Autodesk Inventor part; units mm, degrees
(part 2 of 2)
sketch "Sketch18" plane through (0, 0, 6.35) normal (0, 0, 1) x (1, 0, 0)
  line L0 (518.16, 78.74) -> (525.78, 78.74) construction
  line L1 (525.78, 78.74) -> (525.78, 162.56) construction
  line L2 (525.78, 162.56) -> (518.16, 162.56) construction
  line L3 (518.16, 162.56) -> (518.16, 193.04) construction
  line L4 (518.16, 193.04) -> (525.78, 193.04) construction
  line L5 (525.78, 193.04) -> (525.78, 276.86) construction
  line L6 (525.78, 276.86) -> (518.16, 276.86) construction
  line L7 (518.16, 276.86) -> (518.16, 307.34) construction
  line L8 (518.16, 307.34) -> (525.78, 307.34) construction
  line L9 (525.78, 307.34) -> (525.78, 355.6) construction
  line L10 (525.78, 355.6) -> (464.36, 355.6) construction
  line L11 (464.36, 355.6) -> (464.36, 347.98) construction
  line L12 (464.36, 347.98) -> (436.42, 347.98) construction
  line L13 (436.42, 347.98) -> (436.42, 355.6) construction
  line L14 (436.42, 355.6) -> (276.86, 355.6) construction
  line L15 (276.86, 355.6) -> (276.86, 347.98) construction
  line L16 (276.86, 347.98) -> (248.92, 347.98) construction
  line L17 (248.92, 347.98) -> (248.92, 355.6) construction
  line L18 (248.92, 355.6) -> (89.36, 355.6) construction
  line L19 (89.36, 355.6) -> (89.36, 347.98) construction
  line L20 (89.36, 347.98) -> (61.42, 347.98) construction
  line L21 (61.42, 347.98) -> (61.42, 355.6) construction
  line L22 (61.42, 355.6) -> (0, 355.6) construction
  line L23 (0, 355.6) -> (0, 307.34) construction
  line L24 (0, 307.34) -> (7.62, 307.34) construction
  line L25 (7.62, 307.34) -> (7.62, 276.86) construction
  line L26 (7.62, 276.86) -> (0, 276.86) construction
  line L27 (0, 276.86) -> (0, 193.04) construction
  line L28 (0, 193.04) -> (7.62, 193.04) construction
  line L29 (7.62, 193.04) -> (7.62, 162.56) construction
  line L30 (7.62, 162.56) -> (0, 162.56) construction
  line L31 (0, 162.56) -> (0, 78.74) construction
  line L32 (0, 78.74) -> (7.62, 78.74) construction
  line L33 (7.62, 78.74) -> (7.62, 48.26) construction
  line L34 (7.62, 48.26) -> (0, 48.26) construction
  line L35 (0, 48.26) -> (0, 0) construction
  line L36 (0, 0) -> (7.62, 0) construction
  line L37 (7.62, 0) -> (7.62, -79.375) construction
  line L38 (7.62, -79.375) -> (0, -79.375) construction
  line L39 (0, -79.375) -> (0, -104.775) construction
  line L40 (0, -104.775) -> (7.62, -104.775) construction
  line L41 (7.62, -104.775) -> (7.62, -177.8) construction
  line L42 (7.62, -177.8) -> (50.8, -177.8) construction
  line L43 (50.8, -177.8) -> (50.8, -185.42) construction
  line L44 (50.8, -185.42) -> (76.2, -185.42) construction
  line L45 (76.2, -185.42) -> (76.2, -177.8) construction
  line L46 (76.2, -177.8) -> (177.8, -177.8) construction
  line L47 (177.8, -177.8) -> (177.8, -185.42) construction
  line L48 (177.8, -185.42) -> (203.2, -185.42) construction
  line L49 (203.2, -185.42) -> (203.2, -177.8) construction
  line L50 (203.2, -177.8) -> (242.89, -177.8) construction
  line L51 (242.89, -177.8) -> (242.89, -127.8) construction
  line L52 (242.89, -127.8) -> (282.89, -127.8) construction
  line L53 (282.89, -127.8) -> (282.89, -177.8) construction
  line L54 (282.89, -177.8) -> (322.58, -177.8) construction
  line L55 (322.58, -177.8) -> (322.58, -185.42) construction
  line L56 (322.58, -185.42) -> (347.98, -185.42) construction
  line L57 (347.98, -185.42) -> (347.98, -177.8) construction
  line L58 (347.98, -177.8) -> (449.58, -177.8) construction
  line L59 (449.58, -177.8) -> (449.58, -185.42) construction
  line L60 (449.58, -185.42) -> (474.98, -185.42) construction
  line L61 (474.98, -185.42) -> (474.98, -177.8) construction
  line L62 (474.98, -177.8) -> (518.16, -177.8) construction
  line L63 (518.16, -177.8) -> (518.16, -104.775) construction
  line L64 (518.16, -104.775) -> (525.78, -104.775) construction
  line L65 (525.78, -104.775) -> (525.78, -79.375) construction
  line L66 (525.78, -79.375) -> (518.16, -79.375) construction
  line L67 (518.16, -79.375) -> (518.16, 0) construction
  line L68 (518.16, 0) -> (525.78, 0) construction
  line L69 (525.78, 48.26) -> (525.78, 0) construction
  line L70 (525.78, 48.26) -> (518.16, 48.26) construction
  line L71 (518.16, 48.26) -> (518.16, 78.74) construction
  line L72 (100.076, -104.14) -> (100.076, -73.66) construction
  line L73 (100.076, -73.66) -> (111.506, -73.66) construction
  line L74 (111.506, -73.66) -> (111.506, -104.14) construction
  line L75 (111.506, -104.14) -> (100.076, -104.14) construction
  line L76 (276.86, 7.62) -> (276.86, -1.27) construction
  line L77 (276.86, -1.27) -> (248.92, -1.27) construction
  line L78 (248.92, -1.27) -> (248.92, 7.62) construction
  line L79 (248.92, 7.62) -> (276.86, 7.62) construction
  line L80 (436.42, 24.13) -> (436.42, 33.02) construction
  line L81 (436.42, 33.02) -> (464.36, 33.02) construction
  line L82 (464.36, 33.02) -> (464.36, 24.13) construction
  line L83 (464.36, 24.13) -> (436.42, 24.13) construction
  line L84 (61.42, 24.13) -> (61.42, 33.02) construction
  line L85 (61.42, 33.02) -> (89.36, 33.02) construction
  line L86 (89.36, 33.02) -> (89.36, 24.13) construction
  line L87 (89.36, 24.13) -> (61.42, 24.13) construction
  line L88 (248.92, 176.53) -> (248.92, 185.42) construction
  line L89 (248.92, 185.42) -> (276.86, 185.42) construction
  line L90 (276.86, 185.42) -> (276.86, 176.53) construction
  line L91 (276.86, 176.53) -> (248.92, 176.53) construction
  line L92 (61.42, 176.53) -> (61.42, 185.42) construction
  line L93 (61.42, 185.42) -> (89.36, 185.42) construction
  line L94 (89.36, 185.42) -> (89.36, 176.53) construction
  line L95 (89.36, 176.53) -> (61.42, 176.53) construction
  line L96 (436.42, 176.53) -> (436.42, 185.42) construction
  line L97 (436.42, 185.42) -> (464.36, 185.42) construction
  line L98 (464.36, 185.42) -> (464.36, 176.53) construction
  line L99 (464.36, 176.53) -> (436.42, 176.53) construction
  line L100 (248.92, 24.13) -> (248.92, 33.02) construction
  line L101 (248.92, 33.02) -> (276.86, 33.02) construction
  line L102 (276.86, 33.02) -> (276.86, 24.13) construction
  line L103 (276.86, 24.13) -> (248.92, 24.13) construction
  line L104 (464.36, 7.62) -> (464.36, -1.27) construction
  line L105 (464.36, -1.27) -> (436.42, -1.27) construction
  line L106 (436.42, -1.27) -> (436.42, 7.62) construction
  line L107 (436.42, 7.62) -> (464.36, 7.62) construction
  line L108 (89.36, 7.62) -> (89.36, -1.27) construction
  line L109 (89.36, -1.27) -> (61.42, -1.27) construction
  line L110 (61.42, -1.27) -> (61.42, 7.62) construction
  line L111 (61.42, 7.62) -> (89.36, 7.62) construction
  line L112 (414.02, -104.14) -> (414.02, -73.66) construction
  line L113 (414.02, -73.66) -> (425.45, -73.66) construction
  line L114 (425.45, -73.66) -> (425.45, -104.14) construction
  line L115 (425.45, -104.14) -> (414.02, -104.14) construction
  circle A0 centre (356.64, 267.89) radius 4 construction
  circle A1 centre (356.64, 335.6) radius 4 construction
  circle A2 centre (356.64, 200.18) radius 4 construction
  circle A3 centre (521.97, 24.765) radius 2.25 construction
  circle A4 centre (521.97, 234.95) radius 2.25 construction
  circle A5 centre (3.81, 234.95) radius 2.25 construction
  circle A6 centre (3.81, 24.765) radius 2.25 construction
  circle A7 centre (419.735, -38.1) radius 2.25 construction
  circle A8 centre (105.791, -38.1) radius 2.25 construction
  circle A9 centre (305.84, 3.175) radius 2.25 construction
  circle A10 centre (118.34, 3.175) radius 2.25 construction
  circle A11 centre (305.84, 28.575) radius 2.25 construction
  circle A12 centre (118.34, 28.575) radius 2.25 construction
  circle A13 centre (305.84, 180.975) radius 2.25 construction
  circle A14 centre (118.34, 180.975) radius 2.25 construction
  circle A15 centre (305.84, 352.425) radius 2.25 construction
  circle A16 centre (118.34, 352.425) radius 2.25 construction
  circle A17 centre (219.94, 352.425) radius 2.25 construction
  circle A18 centre (407.44, 352.425) radius 2.25 construction
  circle A19 centre (219.94, 180.975) radius 2.25 construction
  circle A20 centre (407.44, 180.975) radius 2.25 construction
  circle A21 centre (219.94, 28.575) radius 2.25 construction
  circle A22 centre (407.44, 28.575) radius 2.25 construction
  circle A23 centre (219.94, 3.175) radius 2.25 construction
  circle A24 centre (407.44, 3.175) radius 2.25 construction
  circle A25 centre (105.791, -139.7) radius 2.25 construction
  circle A26 centre (419.735, -139.7) radius 2.25 construction
  circle A27 centre (3.81, 120.65) radius 2.25 construction
  circle A28 centre (3.81, 330.835) radius 2.25 construction
  circle A29 centre (521.97, 330.835) radius 2.25 construction
  circle A30 centre (521.97, 120.65) radius 2.25 construction
  line L116 (333.69, -165.1) -> (333.69, -114.3) construction
  line L117 (333.69, -114.3) -> (384.49, -114.3) construction
  line L118 (384.49, -114.3) -> (384.49, -165.1) construction
  line L119 (384.49, -165.1) -> (333.69, -165.1) construction
  line L120 (58.42, -127) -> (58.42, -76.2) construction
  line L121 (58.42, -76.2) -> (83.82, -76.2) construction
  line L122 (83.82, -76.2) -> (83.82, -127) construction
  line L123 (83.82, -127) -> (58.42, -127) construction
  line L124 (467.36, -76.2) -> (467.36, -127) construction
  line L125 (467.36, -127) -> (441.96, -127) construction
  line L126 (441.96, -127) -> (441.96, -76.2) construction
  line L127 (441.96, -76.2) -> (467.36, -76.2) construction
  line L128 (87.1149, 357.8451) -> (251.1651, 357.8451) construction
  line L129 (251.1651, 357.8451) -> (251.1651, 350.2251) construction
  line L130 (251.1651, 350.2251) -> (274.6149, 350.2251) construction
  line L131 (274.6149, 350.2251) -> (274.6149, 357.8451) construction
  line L132 (274.6149, 357.8451) -> (438.6651, 357.8451) construction
  line L133 (438.6651, 357.8451) -> (438.6651, 350.2251) construction
  line L134 (438.6651, 350.2251) -> (462.1149, 350.2251) construction
  line L135 (462.1149, 350.2251) -> (462.1149, 357.8451) construction
  line L136 (462.1149, 357.8451) -> (528.0251, 357.8451) construction
  line L137 (528.0251, 357.8451) -> (528.0251, 305.0949) construction
  line L138 (528.0251, 305.0949) -> (520.4051, 305.0949) construction
  line L139 (520.4051, 305.0949) -> (520.4051, 279.1051) construction
  line L140 (520.4051, 279.1051) -> (528.0251, 279.1051) construction
  line L141 (528.0251, 279.1051) -> (528.0251, 190.7949) construction
  line L142 (528.0251, 190.7949) -> (520.4051, 190.7949) construction
  line L143 (520.4051, 190.7949) -> (520.4051, 164.8051) construction
  line L144 (520.4051, 164.8051) -> (528.0251, 164.8051) construction
  line L145 (528.0251, 164.8051) -> (528.0251, 76.4949) construction
  line L146 (528.0251, 76.4949) -> (520.4051, 76.4949) construction
  line L147 (520.4051, 76.4949) -> (520.4051, 50.5051) construction
  line L148 (520.4051, 50.5051) -> (528.0251, 50.5051) construction
  line L149 (528.0251, 50.5051) -> (528.0251, -2.2451) construction
  line L150 (528.0251, -2.2451) -> (520.4051, -2.2451) construction
  line L151 (520.4051, -2.2451) -> (520.4051, -77.1299) construction
  line L152 (520.4051, -77.1299) -> (528.0251, -77.1299) construction
  line L153 (528.0251, -77.1299) -> (528.0251, -107.0201) construction
  line L154 (528.0251, -107.0201) -> (520.4051, -107.0201) construction
  line L155 (520.4051, -107.0201) -> (520.4051, -180.0451) construction
  line L156 (520.4051, -180.0451) -> (477.2251, -180.0451) construction
  line L157 (477.2251, -180.0451) -> (477.2251, -187.6651) construction
  line L158 (477.2251, -187.6651) -> (447.3349, -187.6651) construction
  line L159 (447.3349, -187.6651) -> (447.3349, -180.0451) construction
  line L160 (447.3349, -180.0451) -> (350.2251, -180.0451) construction
  line L161 (350.2251, -180.0451) -> (350.2251, -187.6651) construction
  line L162 (350.2251, -187.6651) -> (320.3349, -187.6651) construction
  line L163 (320.3349, -187.6651) -> (320.3349, -180.0451) construction
  line L164 (320.3349, -180.0451) -> (280.6449, -180.0451) construction
  line L165 (280.6449, -180.0451) -> (280.6449, -130.0451) construction
  line L166 (280.6449, -130.0451) -> (245.1351, -130.0451) construction
  line L167 (245.1351, -130.0451) -> (245.1351, -180.0451) construction
  line L168 (245.1351, -180.0451) -> (205.4451, -180.0451) construction
  line L169 (205.4451, -180.0451) -> (205.4451, -187.6651) construction
  line L170 (205.4451, -187.6651) -> (175.5549, -187.6651) construction
  line L171 (175.5549, -187.6651) -> (175.5549, -180.0451) construction
  line L172 (175.5549, -180.0451) -> (78.4451, -180.0451) construction
  line L173 (78.4451, -180.0451) -> (78.4451, -187.6651) construction
  line L174 (78.4451, -187.6651) -> (48.5549, -187.6651) construction
  line L175 (48.5549, -187.6651) -> (48.5549, -180.0451) construction
  line L176 (48.5549, -180.0451) -> (5.3749, -180.0451) construction
  line L177 (5.3749, -180.0451) -> (5.3749, -107.0201) construction
  line L178 (5.3749, -107.0201) -> (-2.2451, -107.0201) construction
  line L179 (-2.2451, -107.0201) -> (-2.2451, -77.1299) construction
  line L180 (-2.2451, -77.1299) -> (5.3749, -77.1299) construction
  line L181 (5.3749, -77.1299) -> (5.3749, -2.2451) construction
  line L182 (5.3749, -2.2451) -> (-2.2451, -2.2451) construction
  line L183 (-2.2451, -2.2451) -> (-2.2451, 50.5051) construction
  line L184 (-2.2451, 50.5051) -> (5.3749, 50.5051) construction
  line L185 (5.3749, 50.5051) -> (5.3749, 76.4949) construction
  line L186 (5.3749, 76.4949) -> (-2.2451, 76.4949) construction
  line L187 (-2.2451, 76.4949) -> (-2.2451, 164.8051) construction
  line L188 (-2.2451, 164.8051) -> (5.3749, 164.8051) construction
  line L189 (5.3749, 164.8051) -> (5.3749, 190.7949) construction
  line L190 (5.3749, 190.7949) -> (-2.2451, 190.7949) construction
  line L191 (-2.2451, 190.7949) -> (-2.2451, 279.1051) construction
  line L192 (-2.2451, 279.1051) -> (5.3749, 279.1051) construction
  line L193 (5.3749, 279.1051) -> (5.3749, 305.0949) construction
  line L194 (5.3749, 305.0949) -> (-2.2451, 305.0949) construction
  line L195 (-2.2451, 305.0949) -> (-2.2451, 357.8451) construction
  line L196 (-2.2451, 357.8451) -> (63.6651, 357.8451) construction
  line L197 (63.6651, 357.8451) -> (63.6651, 350.2251) construction
  line L198 (63.6651, 350.2251) -> (87.1149, 350.2251) construction
  line L199 (87.1149, 350.2251) -> (87.1149, 357.8451) construction
  line L200 (61.42, 347.98) -> (89.36, 347.98) projected
  circle A31 centre (63.6651, 350.2251) radius 3.175
  circle A32 centre (87.1149, 350.2251) radius 3.175
  circle A33 centre (251.1651, 350.2251) radius 3.175
  circle A34 centre (274.6149, 350.2251) radius 3.175
  line L201 (464.36, 347.98) -> (436.42, 347.98) projected
  circle A35 centre (438.6651, 350.2251) radius 3.175
  circle A36 centre (462.1149, 350.2251) radius 3.175
  line L202 (518.16, 276.86) -> (518.16, 307.34) projected
  circle A37 centre (520.4051, 305.0949) radius 3.175
  circle A38 centre (520.4051, 279.1051) radius 3.175
  circle A39 centre (520.4051, 190.7949) radius 3.175
  line L203 (525.78, 162.56) -> (518.16, 162.56) projected
  circle A40 centre (520.4051, 164.8051) radius 3.175
  line L204 (518.16, 78.74) -> (525.78, 78.74) projected
  circle A41 centre (520.4051, 76.4949) radius 3.175
  circle A42 centre (520.4051, 50.5051) radius 3.175
  circle A43 centre (520.4051, -2.2451) radius 3.175
  line L205 (525.78, -79.375) -> (518.16, -79.375) projected
  circle A44 centre (520.4051, -77.1299) radius 3.175
  circle A45 centre (520.4051, -107.0201) radius 3.175
  line L206 (474.98, -177.8) -> (518.16, -177.8) projected
  circle A46 centre (477.2251, -180.0451) radius 3.175
  circle A47 centre (447.3349, -180.0451) radius 3.175
  line L207 (347.98, -177.8) -> (449.58, -177.8) projected
  circle A48 centre (350.2251, -180.0451) radius 3.175
  line L208 (322.58, -177.8) -> (322.58, -185.42) projected
  circle A49 centre (320.3349, -180.0451) radius 3.175
  line L209 (203.2, -185.42) -> (203.2, -177.8) projected
  circle A50 centre (205.4451, -180.0451) radius 3.175
  line L210 (177.8, -177.8) -> (177.8, -185.42) projected
  circle A51 centre (175.5549, -180.0451) radius 3.175
  line L211 (76.2, -185.42) -> (76.2, -177.8) projected
  circle A52 centre (78.4451, -180.0451) radius 3.175
  line L212 (7.62, -177.8) -> (50.8, -177.8) projected
  circle A53 centre (48.5549, -180.0451) radius 3.175
  line L213 (0, -104.775) -> (7.62, -104.775) projected
  circle A54 centre (5.3749, -107.0201) radius 3.175
  line L214 (7.62, 0) -> (7.62, -79.375) projected
  circle A55 centre (5.3749, -77.1299) radius 3.175
  line L215 (0, 0) -> (7.62, 0) projected
  circle A56 centre (5.3749, -2.2451) radius 3.175
  circle A57 centre (5.3749, 50.5051) radius 3.175
  circle A58 centre (5.3749, 76.4949) radius 3.175
  circle A59 centre (5.3749, 164.8051) radius 3.175
  line L216 (0, 193.04) -> (7.62, 193.04) projected
  circle A60 centre (5.3749, 190.7949) radius 3.175
  circle A61 centre (5.3749, 279.1051) radius 3.175
  line L217 (7.62, 307.34) -> (7.62, 276.86) projected
  circle A62 centre (5.3749, 305.0949) radius 3.175
  line L218 (87.1149, 183.1749) -> (63.6651, 183.1749) construction
  line L219 (63.6651, 183.1749) -> (63.6651, 178.7751) construction
  line L220 (63.6651, 178.7751) -> (87.1149, 178.7751) construction
  line L221 (87.1149, 178.7751) -> (87.1149, 183.1749) construction
  line L222 (274.6149, 183.1749) -> (251.1651, 183.1749) construction
  line L223 (251.1651, 183.1749) -> (251.1651, 178.7751) construction
  line L224 (251.1651, 178.7751) -> (274.6149, 178.7751) construction
  line L225 (274.6149, 178.7751) -> (274.6149, 183.1749) construction
  line L226 (462.1149, 183.1749) -> (438.6651, 183.1749) construction
  line L227 (438.6651, 183.1749) -> (438.6651, 178.7751) construction
  line L228 (438.6651, 178.7751) -> (462.1149, 178.7751) construction
  line L229 (462.1149, 178.7751) -> (462.1149, 183.1749) construction
  line L230 (462.1149, 30.7749) -> (438.6651, 30.7749) construction
  line L231 (438.6651, 30.7749) -> (438.6651, 26.3751) construction
  line L232 (438.6651, 26.3751) -> (462.1149, 26.3751) construction
  line L233 (462.1149, 26.3751) -> (462.1149, 30.7749) construction
  line L234 (462.1149, 5.3749) -> (462.1149, 0.9751) construction
  line L235 (462.1149, 0.9751) -> (438.6651, 0.9751) construction
  line L236 (438.6651, 0.9751) -> (438.6651, 5.3749) construction
  line L237 (438.6651, 5.3749) -> (462.1149, 5.3749) construction
  line L238 (274.6149, 5.3749) -> (274.6149, 0.9751) construction
  line L239 (274.6149, 0.9751) -> (251.1651, 0.9751) construction
  line L240 (251.1651, 0.9751) -> (251.1651, 5.3749) construction
  line L241 (251.1651, 5.3749) -> (274.6149, 5.3749) construction
  line L242 (274.6149, 30.7749) -> (251.1651, 30.7749) construction
  line L243 (251.1651, 30.7749) -> (251.1651, 26.3751) construction
  line L244 (251.1651, 26.3751) -> (274.6149, 26.3751) construction
  line L245 (274.6149, 26.3751) -> (274.6149, 30.7749) construction
  line L246 (87.1149, 5.3749) -> (87.1149, 0.9751) construction
  line L247 (87.1149, 0.9751) -> (63.6651, 0.9751) construction
  line L248 (63.6651, 0.9751) -> (63.6651, 5.3749) construction
  line L249 (63.6651, 5.3749) -> (87.1149, 5.3749) construction
  line L250 (87.1149, 30.7749) -> (63.6651, 30.7749) construction
  line L251 (63.6651, 30.7749) -> (63.6651, 26.3751) construction
  line L252 (63.6651, 26.3751) -> (87.1149, 26.3751) construction
  line L253 (87.1149, 26.3751) -> (87.1149, 30.7749) construction
  line L254 (102.3211, -75.9051) -> (102.3211, -101.8949) construction
  line L255 (102.3211, -101.8949) -> (109.2609, -101.8949) construction
  line L256 (109.2609, -101.8949) -> (109.2609, -75.9051) construction
  line L257 (109.2609, -75.9051) -> (102.3211, -75.9051) construction
  line L258 (416.2651, -75.9051) -> (416.2651, -101.8949) construction
  line L259 (416.2651, -101.8949) -> (423.2049, -101.8949) construction
  line L260 (423.2049, -101.8949) -> (423.2049, -75.9051) construction
  line L261 (423.2049, -75.9051) -> (416.2651, -75.9051) construction
  circle A63 centre (63.6651, 183.1749) radius 3.175
  line L262 (89.36, 185.42) -> (61.42, 185.42) projected
  circle A64 centre (87.1149, 183.1749) radius 3.175
  line L263 (89.36, 176.53) -> (89.36, 185.42) projected
  circle A65 centre (87.1149, 178.7751) radius 3.175
  line L264 (89.36, 176.53) -> (61.42, 176.53) projected
  circle A66 centre (63.6651, 178.7751) radius 3.175
  circle A67 centre (251.1651, 183.1749) radius 3.175
  circle A68 centre (251.1651, 178.7751) radius 3.175
  circle A69 centre (274.6149, 178.7751) radius 3.175
  line L265 (276.86, 185.42) -> (276.86, 176.53) projected
  circle A70 centre (274.6149, 183.1749) radius 3.175
  line L266 (464.36, 185.42) -> (436.42, 185.42) projected
  circle A71 centre (438.6651, 183.1749) radius 3.175
  circle A72 centre (438.6651, 178.7751) radius 3.175
  line L267 (464.36, 176.53) -> (436.42, 176.53) projected
  circle A73 centre (462.1149, 178.7751) radius 3.175
  circle A74 centre (462.1149, 183.1749) radius 3.175
  circle A75 centre (438.6651, 30.7749) radius 3.175
  line L268 (436.42, 24.13) -> (436.42, 33.02) projected
  circle A76 centre (438.6651, 26.3751) radius 3.175
  circle A77 centre (462.1149, 26.3751) radius 3.175
  circle A78 centre (462.1149, 30.7749) radius 3.175
  circle A79 centre (462.1149, 5.3749) radius 3.175
  circle A80 centre (462.1149, 0.9751) radius 3.175
  circle A81 centre (438.6651, 0.9751) radius 3.175
  line L269 (436.42, -1.27) -> (436.42, 7.62) projected
  circle A82 centre (438.6651, 5.3749) radius 3.175
  circle A83 centre (274.6149, 0.9751) radius 3.175
  circle A84 centre (274.6149, 5.3749) radius 3.175
  circle A85 centre (251.1651, 5.3749) radius 3.175
  line L270 (248.92, -1.27) -> (248.92, 7.62) projected
  circle A86 centre (251.1651, 0.9751) radius 3.175
  line L271 (276.86, 33.02) -> (276.86, 24.13) projected
  circle A87 centre (274.6149, 26.3751) radius 3.175
  circle A88 centre (274.6149, 30.7749) radius 3.175
  circle A89 centre (251.1651, 30.7749) radius 3.175
  circle A90 centre (251.1651, 26.3751) radius 3.175
  circle A91 centre (87.1149, 30.7749) radius 3.175
  circle A92 centre (87.1149, 26.3751) radius 3.175
  circle A93 centre (63.6651, 26.3751) radius 3.175
  circle A94 centre (63.6651, 30.7749) radius 3.175
  circle A95 centre (63.6651, 5.3749) radius 3.175
  line L272 (61.42, 7.62) -> (61.42, -1.27) projected
  circle A96 centre (63.6651, 0.9751) radius 3.175
  line L273 (89.36, -1.27) -> (61.42, -1.27) projected
  circle A97 centre (87.1149, 0.9751) radius 3.175
  line L274 (89.36, 7.62) -> (89.36, -1.27) projected
  circle A98 centre (87.1149, 5.3749) radius 3.175
  circle A99 centre (102.3211, -75.9051) radius 3.175
  line L275 (111.506, -73.66) -> (111.506, -104.14) projected
  circle A100 centre (109.2609, -75.9051) radius 3.175
  circle A101 centre (109.2609, -101.8949) radius 3.175
  circle A102 centre (102.3211, -101.8949) radius 3.175
  circle A103 centre (416.2651, -101.8949) radius 3.175
  line L276 (425.45, -104.14) -> (414.02, -104.14) projected
  circle A104 centre (423.2049, -101.8949) radius 3.175
  circle A105 centre (423.2049, -75.9051) radius 3.175
  circle A106 centre (416.2651, -75.9051) radius 3.175
  dimension "d174" = 6.35
  dimension "d175" = 6.35
  dimension "d176" = 6.35
  dimension "d177" = 6.35
  dimension "d178" = 6.35
  dimension "d179" = 6.35
  dimension "d180" = 6.35
  dimension "d181" = 6.35
  dimension "d182" = 6.35
  dimension "d183" = 6.35
  dimension "d184" = 6.35
  dimension "d185" = 6.35
  constraints: 232 end point, 76 coincident, 332 other
extrude "Extrusion18" cut sketch "Sketch18" along normal through all both and the other way through all contours A31 L200 | L200 A31 | A32 L200 | L200 A32 | A33 | A34 | A36 L201 | L201 A36 | A35 L201 | L201 A35 | A38 L202 | L202 A38 | A37 L202 | L202 A37 | A39 | A40 L203 | L203 A40 | A41 L204 | L204 A41 | A42 | A43 | A44 L205 | L205 A44 | A45 | A46 L206 | L206 A46 | A47 L207 | L207 A47 | A48 L207 | L207 A48 | A49 L208 | L208 A49 | A50 L209 | L209 A50 | A51 L210 | L210 A51 | A52 L211 | L211 A52 | A53 L212 | L212 A53 | A54 L213 | L213 A54 | A56 L214 | L214 A56 L215 | L215 A56 | A55 L214 | L214 A55 | A57 | A58 | A59 | A60 L216 | L216 A60 | L217 A61 | A61 L217 | A62 L217 | L217 A62 | A63 A66 L262 | L262 A63 | A66 L264 A63 | A63 A66 | A64 L262 | L262 L263 A65 A64 | A64 A65 L263 | A65 L263 A64 | A64 L263 L264 A65 | L264 A66 | A65 A64 L263 | A64 A65 L263 | L264 A65 | A67 A68 | A68 A67 | A67 A68 | L265 A70 A69 | A69 A70 L265 | A70 L265 A69 | A69 L265 A70 | L265 A69 A70 | A69 L265 A70 | A74 A73 L266 | L266 A74 | A71 A72 L266 | L266 A71 | A74 A73 L267 | A73 A74 | L267 A73 | A72 A71 | A71 A72 L267 | A72 L267 | A75 A76 L268 | L268 A76 A75 | A76 L268 A75 | A75 L268 A76 | A76 L268 A75 | A75 L268 A76 | A77 A78 | A78 A77 | A77 A78 | A79 A80 | A80 A79 | A79 A80 | L269 A82 A81 | A81 A82 L269 | A82 L269 A81 | A81 L269 A82 | L269 A81 A82 | A81 L269 A82 | A83 A84 | A84 A83 | A83 A84 | A85 A86 L270 | L270 A86 A85 | A86 L270 A85 | A85 L270 A86 | A86 L270 A85 | A85 L270 A86 | A88 A87 L271 | L271 A87 A88 | A87 A88 L271 | L271 A88 A87 | A88 L271 A87 | A88 A87 L271 | A89 A90 | A90 A89 | A89 A90 | A91 A92 | A92 A91 | A91 A92 | A93 A94 | A94 A93 | A93 A94 | A95 A96 L272 | L272 A96 A95 | A96 L273 L272 A95 | A95 L272 A96 | A96 L272 A95 | A95 L272 A96 | L273 A96 | A97 L273 | L274 A98 A97 | L273 A97 A98 L274 | A98 A97 L274 | L274 A97 A98 | A98 L274 A97 | A97 L274 A98 | A99 | A100 L275 | L275 A100 | A101 L275 | L275 A101 | A102 | A103 L276 | L276 A103 | A104 L276 | L276 A104 | A105 | A106
equation "\"d2\" = Panel_Thickness"
equation "\"d4\" = Panel_Thickness + Fit_Tolerance"
equation "\"d5\" = Panel_Thickness + Fit_Tolerance"
equation "\"d7\" = d6"
equation "\"d8\" = d6"
equation "\"d10\" = d9"
equation "\"d14\" = Panel_Thickness"
equation "\"d24\" = Panel_Thickness"
equation "\"d27\" = Panel_Thickness + Fit_Tolerance"
equation "\"d36\" = Panel_Thickness"
equation "\"d38\" = Panel_Thickness + Fit_Tolerance"
equation "\"d39\" = Panel_Thickness"
equation "\"d46\" = Panel_Thickness"
equation "\"d56\" = Panel_Thickness"
equation "\"d60\" = Panel_Thickness"
equation "\"d66\" = Panel_Thickness"
equation "\"d68\" = Panel_Thickness"
equation "\"d70\" = Fit_Tolerance"
equation "\"d71\" = Fit_Tolerance"
equation "\"d72\" = Fit_Tolerance"
equation "\"d73\" = Panel_Thickness"
equation "\"d77\" = Panel_Thickness"
equation "\"d90\" = Panel_Thickness"
equation "\"d94\" = Panel_Thickness"
equation "\"d96\" = Panel_Thickness"
equation "\"d104\" = Panel_Thickness"
equation "\"d111\" = 0.5 * Panel_Thickness"
equation "\"d153\" = Fit_Tolerance"
equation "\"d154\" = Fit_Tolerance"
equation "\"d155\" = Fit_Tolerance"
equation "\"d156\" = Fit_Tolerance"
equation "\"d157\" = Fit_Tolerance"
equation "\"d158\" = Fit_Tolerance"
equation "\"d159\" = Fit_Tolerance"
equation "\"d161\" = Fit_Tolerance"
equation "\"d162\" = Fit_Tolerance"
equation "\"d163\" = Fit_Tolerance"
equation "\"d164\" = Fit_Tolerance"
equation "\"d165\" = Fit_Tolerance"
equation "\"d166\" = Fit_Tolerance"
equation "\"d167\" = Fit_Tolerance"
equation "\"d168\" = Fit_Tolerance"
equation "\"d169\" = Fit_Tolerance"
equation "\"d170\" = Fit_Tolerance"
equation "\"d171\" = Fit_Tolerance"
equation "\"d174\" = Tool_Dia"
equation "\"d175\" = d174"
equation "\"d176\" = d174"
equation "\"d177\" = d176"
equation "\"d178\" = d177"
equation "\"d179\" = d178"
equation "\"d180\" = d175"
equation "\"d181\" = d180"
equation "\"d182\" = d179"
equation "\"d183\" = d178"
equation "\"d184\" = d183"
equation "\"d185\" = d181"
equation "\"Panel_Thickness\" = 6.35"
equation "\"Fit_Tolerance\" = 1.27"
equation "\"Tool_Dia\" = 6.35"
body "Solid1"
